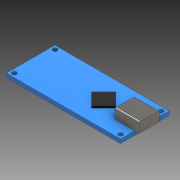
# Autodesk Inventor part: MICROCONTROLLER
Saved by Autodesk Inventor 2017 (Build 210142000, 142)
## iProperties
Created: 2017-04-01
Part Number: MICROCONTROLLER
Material: Generic
Document SubType Name: Modeling
Designer: Muchen
Density: 1 g/cm^3
Appearance: Default
Author: Muchen
Autodesk Inventor part; units mm, degrees
ref_plane "YZ Plane" through (0, 0, 0) normal (1, 0, 0) x (0, 1, 0)
ref_plane "XZ Plane" through (0, 0, 0) normal (0, 1, 0) x (-1, 0, 0)
ref_plane "XY Plane" through (0, 0, 0) normal (0, 0, 1) x (1, 0, 0)
sketch "Sketch1" plane through (0, 0, 0) normal (0, 0, 1) x (1, 0, 0)
  line L0 (0, 0) -> (43.38, 0)
  line L1 (43.38, 0) -> (43.38, 18.44)
  line L2 (43.38, 18.44) -> (0, 18.44)
  line L3 (0, 18.44) -> (0, 0)
  circle A0 centre (1.5, 16.94) radius 0.85
  circle A1 centre (1.5, 1.5) radius 0.85
  circle A2 centre (41.88, 16.94) radius 0.85
  circle A3 centre (41.88, 1.5) radius 0.85
  dimension "d0" = 43.38
  dimension "d1" = 18.44
  dimension "d2" = 1.7
  dimension "d3" = 1.5
  dimension "d4" = 1.5
  dimension "d5" = 1.5
  dimension "d6" = 1.5
  constraints: 8 end point, 4 centre point, 3 equal radius, 2 horizontal alignment, 2 parallel, 2 vertical alignment, 1 horizontal, 1 perpendicular
  measures "d0" distance of L2.end L1.end
  measures "d1" distance of L2.end L0.start
  measures "d2" diameter of A1
  measures "d3" distance from line of L2 A0.centre
  measures "d4" distance from line of L0 A1.centre
  measures "d5" distance from line of L3 A0.centre
  measures "d6" distance from line of L1 A2.centre
extrude "Extrusion1" add sketch "Sketch1" along normal blind 1.53
sketch "Sketch2" plane through (0, 0, 1.53) normal (0, 0, 1) x (1, 0, 0)
  line L0 (23.1338, 9.22) -> (27.73, 13.8162)
  line L1 (27.73, 13.8162) -> (32.3262, 9.22)
  line L2 (32.3262, 9.22) -> (27.73, 4.6238)
  line L3 (27.73, 4.6238) -> (23.1338, 9.22)
  line L4 (0, 0) -> (43.38, 0) projected
  line L5 (0, 18.44) -> (0, 0) projected
  line L6 (43.38, 0) -> (43.38, 18.44) projected
  line L7 (35.86, 5.42) -> (45.11, 5.42)
  line L8 (45.11, 5.42) -> (45.11, 13.02)
  line L9 (45.11, 13.02) -> (35.86, 13.02)
  line L10 (35.86, 13.02) -> (35.86, 5.42)
  point P0 (0, 9.22)
  point P1 (45.11, 9.22)
  dimension "d9" = 45
  dimension "d10" = 6.5
  dimension "d11" = 15.65
  dimension "d12" = 9.25
  dimension "d13" = 7.6
  dimension "d14" = 1.73
  constraints: 16 end point, 4 parallel, 3 perpendicular, 2 horizontal alignment, 2 midpoint, 1 horizontal
  measures "d9" angle of L4 L2
  measures "d10" distance of L2.end L0.start
  measures "d11" distance from line of L6 L0.end
  measures "d12" distance of L8.end L9.end
  measures "d13" distance of L7.end L8.end
  measures "d14" distance between parallel lines of L6 L8
extrude "Extrusion2" add sketch "Sketch2" along normal blind 3.75 contours L7 L10 L9 L6 | L6 L9 L8 L7
extrude "Extrusion3" add sketch "Sketch2" along normal blind 0.8 contours L0 L1 L2 L3
fillet "Fillet1" radius 0.5 2 edges at (40.485, 5.42, 5.28) (40.485, 13.02, 5.28)
body "Solid1"
